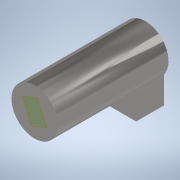
# Autodesk Inventor part: motor jaws
Saved by Autodesk Inventor 2020 (Build 240168000, 168)
## iProperties
Created: 2020-07-02
Part Number: motor jaws
Material: Generic
Document SubType Name: Sheet Metal
Designer: Ashiqrahman
Density: 1 g/cm^3
Sheet Metal Rule: Default
Appearance: Knurled 45
Author: Ashiqrahman
Autodesk Inventor part; units mm, degrees
ref_plane "YZ Plane" through (0, 0, 0) normal (1, 0, 0) x (0, 1, 0)
ref_plane "XZ Plane" through (0, 0, 0) normal (0, 1, 0) x (-1, 0, 0)
ref_plane "XY Plane" through (0, 0, 0) normal (0, 0, 1) x (1, 0, 0)
ref_plane "Work Plane1" through (67.2859, -5.594, 25.8909) normal (0, 0, -1) x (0.9284, 0.3715, 0)
sketch "Sketch2" plane through (67.2859, -5.594, 25.8909) normal (0, 0, -1) x (0.9284, 0.3715, 0)
  circle A0 centre (0, 0) radius 12.5
  point P0 (-60.3924, -30.19)
  dimension "d0" = 25
  constraints: 1 centre point
  measures "d0" diameter of A0
extrude "Extrusion1" add sketch "Sketch2" along normal blind 60
sketch "Sketch3" plane through (67.2859, -5.594, -34.1091) normal (0, 0, -1) x (-1, 0, 0)
  circle A0 centre (0, 0) radius 12.5 projected
  line L0 (10, -22) -> (10, 8) projected
  line L1 (-10, -22) -> (-10, 8) projected
  line L2 (-30, -22) -> (10, -22) projected
  point P0 (67.2859, 5.594)
  point P1 (10, -7.5)
  point P2 (-10, -7.5)
extrude "Extrusion2" add sketch "Sketch3" against normal blind 15 contours L0 L2 L1 A0
equation "\"BendRadius\" = Thickness"
equation "\"BendReliefWidth\" = Thickness"
equation "\"BendReliefDepth\" = 0.5 * Thickness"
equation "\"CornerReliefSize\" = 4 * Thickness"
equation "\"MinimumRemnant\" = 2 * Thickness"
equation "\"TransitionRadius\" = BendRadius"
equation "\"JacobiRadiusSize\" = Thickness"
equation "\"GapSize\" = Thickness"
equation "\"Thickness\" = 0.5"
body "Solid1"
